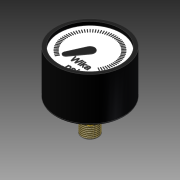
# Autodesk Inventor part: 9690242
Saved by Autodesk Inventor 2014 SP1 (Build 180222100, 222)
## iProperties
Category: Pneumatics
Shininess: 64.0
Length Units: 11269
Angle Units: 11279
Time Units: 11290
Mass Units: 11283
Length Display Precision: 3
Angle Display Precision: 2
Compacted: True
Part Number: 9690242
Document SubType Name: Modeling
Created: 2005-01-09
Manufacturer: Standard
Standards Organization: Custom
Catalog Web Link: www.wika.com
Description: Pressure Gauge
Vendor: WIKA
Density: 1 g/cm^3
Project: FIRST
Material: Generic
Appearance: Glossy - Black
Mass: 32.8384 g
Surface Area: 68.6686 cm^2
Volume: 32.8384 cm^3
Density: 0.0
Volumn: 0.0
Area: 0.0
PropertySet Name: Model Information
Control State: 0
Master: False
Checked Out: False
Title: Pressure Gauge
Author: Autodesk, Inc.
Autodesk Inventor part; units mm, degrees
ref_plane "YZ Plane" through (0, 0, 0) normal (1, 0, 0) x (0, 1, 0)
ref_plane "XZ Plane" through (0, 0, 0) normal (0, 1, 0) x (-1, 0, 0)
ref_plane "XY Plane" through (0, 0, 0) normal (0, 0, 1) x (1, 0, 0)
sketch "Sketch13" plane through (0, 0, 0) normal (0, 0, 1) x (1, 0, 0)
  circle A0 centre (0, 0) radius 20
  dimension "d46" = 40
  constraints: 1 centre point, 1 coincident
  measures "d46" diameter of A0
extrude "Extrusion13" add sketch "Sketch13" along normal blind 26
sketch "Sketch15" plane through (0, 0, 0) normal (0, 0, -1) x (-1, 0, 0)
  line L0 (-7, 7) -> (7, 7)
  line L1 (7, 7) -> (7, -7)
  line L2 (7, -7) -> (-7, -7)
  line L3 (-7, -7) -> (-7, 7)
  line L4 (-28, 0) -> (28, 0) projected
  line L5 (0, -28) -> (0, 28) projected
  dimension "d52" = 14
  dimension "d53" = 14
  constraints: 8 end point, 2 parallel, 1 horizontal, 1 perpendicular, 2 other
  measures "d52" distance of L2.end L0.start
  measures "d53" distance of L0.start L0.end
extrude "Extrusion15" add sketch "Sketch15" along normal blind 8
sketch "Sketch16" plane through (0, 0, -8) normal (0, 0, -1) x (-1, 0, 0)
  circle A0 centre (0, 0) radius 4.7625
  dimension "d58" = 9.525
  constraints: 1 centre point, 1 coincident
  measures "d58" diameter of A0
extrude "Extrusion16" add sketch "Sketch16" along normal blind 10
thread "Thread3" size "1/8" designation "1/8 - 27 NPT" standard "NPT" full length
sketch "Sketch18" plane through (0, 0, 26) normal (0, 0, 1) x (1, 0, 0)
  circle A0 centre (0, 0) radius 20 projected
  circle A1 centre (0, 0) radius 18
  dimension "d66" = 2
  constraints: 1 centre point
  measures "d66" radial gap between concentric circles of A0 A1
extrude "Extrusion18" cut sketch "Sketch18" against normal blind 2 contours A1
sketch "Sketch20" plane through (0, 0, -18) normal (0, 0, -1) x (-1, 0, 0)
  circle A0 centre (0, 0) radius 4.7625 projected
  circle A1 centre (0, 0) radius 1.5
  dimension "d75" = 3
  constraints: 1 centre point, 1 coincident
  measures "d75" diameter of A1
extrude "Extrusion19" cut sketch "Sketch20" against normal blind 10 contours A1
sketch "Sketch19" plane through (0, 0, 24) normal (0, 0, 1) x (1, 0, 0)
  line L0 (-6.3869, -7.2966) -> (14.5094, -7.2966) construction
  line L1 (14.5094, -7.2966) -> (14.5094, -16.6783) construction
  line L2 (14.5094, -16.6783) -> (-6.3869, -16.6783) construction
  line L3 (-6.3869, -16.6783) -> (-6.3869, -7.2966) construction
  circle A0 centre (0, 0) radius 18 projected
  circle A1 centre (0, 0) radius 15 construction
  line L4 (0, 0) -> (-6.5, -11.2583) construction
  line L5 (0, 0) -> (15, 0) construction
  line L6 (-7.6083, -12.9279) -> (-6.6083, -11.1958)
  line L7 (-6.6083, -11.1958) -> (-6.3917, -11.3208)
  line L8 (-6.3917, -11.3208) -> (-7.3917, -13.0529)
  line L9 (-7.3917, -13.0529) -> (-7.6083, -12.9279)
  line L10 (-8.6155, -12.2796) -> (-7.4805, -10.6329)
  line L11 (-7.4805, -10.6329) -> (-7.2746, -10.7748)
  line L12 (-7.2746, -10.7748) -> (-8.4096, -12.4215)
  line L13 (-8.4096, -12.4215) -> (-8.6155, -12.2796)
  line L14 (-9.5677, -11.5531) -> (-8.305, -10.0022)
  line L15 (-8.305, -10.0022) -> (-8.1111, -10.16)
  line L16 (-8.1111, -10.16) -> (-9.3739, -11.7109)
  line L17 (-9.3739, -11.7109) -> (-9.5677, -11.5531)
  line L18 (-10.459, -10.7529) -> (-9.0765, -9.3076)
  line L19 (-9.0765, -9.3076) -> (-8.8959, -9.4805)
  line L20 (-8.8959, -9.4805) -> (-10.2784, -10.9257)
  line L21 (-10.2784, -10.9257) -> (-10.459, -10.7529)
  line L22 (-11.2836, -9.8841) -> (-9.7902, -8.5538)
  line L23 (-9.7902, -8.5538) -> (-9.6239, -8.7405)
  line L24 (-9.6239, -8.7405) -> (-11.1173, -10.0708)
  line L25 (-11.1173, -10.0708) -> (-11.2836, -9.8841)
  line L26 (-12.0362, -8.9523) -> (-10.4415, -7.7454)
  line L27 (-10.4415, -7.7454) -> (-10.2906, -7.9448)
  line L28 (-10.2906, -7.9448) -> (-11.8854, -9.1517)
  line L29 (-11.8854, -9.1517) -> (-12.0362, -8.9523)
  line L30 (-12.7121, -7.9635) -> (-11.0262, -6.8876)
  line L31 (-11.0262, -6.8876) -> (-10.8917, -7.0984)
  line L32 (-10.8917, -7.0984) -> (-12.5777, -8.1742)
  line L33 (-12.5777, -8.1742) -> (-12.7121, -7.9635)
  line L34 (-13.307, -6.9238) -> (-11.5405, -5.9859)
  line L35 (-11.5405, -5.9859) -> (-11.4233, -6.2067)
  line L36 (-11.4233, -6.2067) -> (-13.1898, -7.1446)
  line L37 (-13.1898, -7.1446) -> (-13.307, -6.9238)
  line L38 (-13.817, -5.84) -> (-11.9813, -5.0461)
  line L39 (-11.9813, -5.0461) -> (-11.8821, -5.2755)
  line L40 (-11.8821, -5.2755) -> (-13.7178, -6.0695)
  line L41 (-13.7178, -6.0695) -> (-13.817, -5.84)
  line L42 (-14.2389, -4.719) -> (-12.3458, -4.074)
  line L43 (-12.3458, -4.074) -> (-12.2651, -4.3107)
  line L44 (-12.2651, -4.3107) -> (-14.1583, -4.9557)
  line L45 (-14.1583, -4.9557) -> (-14.2389, -4.719)
  line L46 (-14.57, -3.5679) -> (-12.6315, -3.076)
  line L47 (-12.6315, -3.076) -> (-12.57, -3.3184)
  line L48 (-12.57, -3.3184) -> (-14.5085, -3.8102)
  line L49 (-14.5085, -3.8102) -> (-14.57, -3.5679)
  line L50 (-14.8082, -2.3941) -> (-12.8366, -2.0584)
  line L51 (-12.8366, -2.0584) -> (-12.7947, -2.3049)
  line L52 (-12.7947, -2.3049) -> (-14.7663, -2.6405)
  line L53 (-14.7663, -2.6405) -> (-14.8082, -2.3941)
  line L54 (-14.952, -1.2049) -> (-12.9599, -1.0277)
  line L55 (-12.9599, -1.0277) -> (-12.9378, -1.2767)
  line L56 (-12.9378, -1.2767) -> (-14.9299, -1.4539)
  line L57 (-14.9299, -1.4539) -> (-14.952, -1.2049)
  line L58 (-15.0005, -0.0081) -> (-13.0006, 0.0096)
  line L59 (-13.0006, 0.0096) -> (-12.9984, -0.2404)
  line L60 (-12.9984, -0.2404) -> (-14.9983, -0.2581)
  line L61 (-14.9983, -0.2581) -> (-15.0005, -0.0081)
  line L62 (-14.9533, 1.1887) -> (-12.9584, 1.0469)
  line L63 (-12.9584, 1.0469) -> (-12.9761, 0.7975)
  line L64 (-12.9761, 0.7975) -> (-14.9711, 0.9394)
  line L65 (-14.9711, 0.9394) -> (-14.9533, 1.1887)
  line L66 (-14.8108, 2.378) -> (-12.8335, 2.0774)
  line L67 (-12.8335, 2.0774) -> (-12.8711, 1.8303)
  line L68 (-12.8711, 1.8303) -> (-14.8484, 2.1309)
  line L69 (-14.8484, 2.1309) -> (-14.8108, 2.378)
  line L70 (-14.5739, 3.5521) -> (-12.6269, 3.0947)
  line L71 (-12.6269, 3.0947) -> (-12.6841, 2.8514)
  line L72 (-12.6841, 2.8514) -> (-14.6311, 3.3088)
  line L73 (-14.6311, 3.3088) -> (-14.5739, 3.5521)
  line L74 (-14.244, 4.7036) -> (-12.3397, 4.0923)
  line L75 (-12.3397, 4.0923) -> (-12.4161, 3.8543)
  line L76 (-12.4161, 3.8543) -> (-14.3204, 4.4656)
  line L77 (-14.3204, 4.4656) -> (-14.244, 4.7036)
  line L78 (-13.8233, 5.8251) -> (-11.9739, 5.0638)
  line L79 (-11.9739, 5.0638) -> (-12.069, 4.8326)
  line L80 (-12.069, 4.8326) -> (-13.9185, 5.5939)
  line L81 (-13.9185, 5.5939) -> (-13.8233, 5.8251)
  line L82 (-13.3145, 6.9094) -> (-11.5317, 6.003)
  line L83 (-11.5317, 6.003) -> (-11.645, 5.7802)
  line L84 (-11.645, 5.7802) -> (-13.4278, 6.6866)
  line L85 (-13.4278, 6.6866) -> (-13.3145, 6.9094)
  line L86 (-12.7208, 7.9497) -> (-11.0159, 6.904)
  line L87 (-11.0159, 6.904) -> (-11.1467, 6.6908)
  line L88 (-11.1467, 6.6908) -> (-12.8515, 7.7366)
  line L89 (-12.8515, 7.7366) -> (-12.7208, 7.9497)
  line L90 (-12.0459, 8.9393) -> (-10.43, 7.7609)
  line L91 (-10.43, 7.7609) -> (-10.5773, 7.5589)
  line L92 (-10.5773, 7.5589) -> (-12.1932, 8.7373)
  line L93 (-12.1932, 8.7373) -> (-12.0459, 8.9393)
  line L94 (-11.2943, 9.8719) -> (-9.7775, 8.5683)
  line L95 (-9.7775, 8.5683) -> (-9.9405, 8.3787)
  line L96 (-9.9405, 8.3787) -> (-11.4573, 9.6823)
  line L97 (-11.4573, 9.6823) -> (-11.2943, 9.8719)
  line L98 (-10.4707, 10.7416) -> (-9.0627, 9.3211)
  line L99 (-9.0627, 9.3211) -> (-9.2403, 9.1451)
  line L100 (-9.2403, 9.1451) -> (-10.6482, 10.5656)
  line L101 (-10.6482, 10.5656) -> (-10.4707, 10.7416)
  line L102 (-9.5802, 11.5427) -> (-8.2901, 10.0144)
  line L103 (-8.2901, 10.0144) -> (-8.4812, 9.8532)
  line L104 (-8.4812, 9.8532) -> (-9.7713, 11.3815)
  line L105 (-9.7713, 11.3815) -> (-9.5802, 11.5427)
  line L106 (-8.6288, 12.2703) -> (-7.4647, 10.644)
  line L107 (-7.4647, 10.644) -> (-7.668, 10.4985)
  line L108 (-7.668, 10.4985) -> (-8.832, 12.1248)
  line L109 (-8.832, 12.1248) -> (-8.6288, 12.2703)
  line L110 (-7.6222, 12.9196) -> (-6.5917, 11.2056)
  line L111 (-6.5917, 11.2056) -> (-6.8059, 11.0768)
  line L112 (-6.8059, 11.0768) -> (-7.8365, 12.7908)
  line L113 (-7.8365, 12.7908) -> (-7.6222, 12.9196)
  line L114 (-6.5671, 13.4866) -> (-5.6766, 11.6958)
  line L115 (-5.6766, 11.6958) -> (-5.9004, 11.5845)
  line L116 (-5.9004, 11.5845) -> (-6.791, 13.3753)
  line L117 (-6.791, 13.3753) -> (-6.5671, 13.4866)
  line L118 (-5.4702, 13.9676) -> (-4.7253, 12.1114)
  line L119 (-4.7253, 12.1114) -> (-4.9574, 12.0183)
  line L120 (-4.9574, 12.0183) -> (-5.7022, 13.8745)
  line L121 (-5.7022, 13.8745) -> (-5.4702, 13.9676)
  line L122 (-4.3383, 14.3595) -> (-3.744, 12.4498)
  line L123 (-3.744, 12.4498) -> (-3.9827, 12.3755)
  line L124 (-3.9827, 12.3755) -> (-4.577, 14.2852)
  line L125 (-4.577, 14.2852) -> (-4.3383, 14.3595)
  line L126 (-3.1788, 14.6598) -> (-2.7387, 12.7089)
  line L127 (-2.7387, 12.7089) -> (-2.9826, 12.6539)
  line L128 (-2.9826, 12.6539) -> (-3.4227, 14.6048)
  line L129 (-3.4227, 14.6048) -> (-3.1788, 14.6598)
  line L130 (-1.999, 14.8667) -> (-1.716, 12.8869)
  line L131 (-1.716, 12.8869) -> (-1.9635, 12.8515)
  line L132 (-1.9635, 12.8515) -> (-2.2465, 14.8313)
  line L133 (-2.2465, 14.8313) -> (-1.999, 14.8667)
  line L134 (-0.8065, 14.9788) -> (-0.6823, 12.9827)
  line L135 (-0.6823, 12.9827) -> (-0.9318, 12.9672)
  line L136 (-0.9318, 12.9672) -> (-1.056, 14.9633)
  line L137 (-1.056, 14.9633) -> (-0.8065, 14.9788)
  line L138 (0.3912, 14.9954) -> (0.3557, 12.9957)
  line L139 (0.3557, 12.9957) -> (0.1057, 13.0002)
  line L140 (0.1057, 13.0002) -> (0.1412, 14.9999)
  line L141 (0.1412, 14.9999) -> (0.3912, 14.9954)
  line L142 (1.5864, 14.9164) -> (1.3915, 12.9259)
  line L143 (1.3915, 12.9259) -> (1.1426, 12.9503)
  line L144 (1.1426, 12.9503) -> (1.3376, 14.9408)
  line L145 (1.3376, 14.9408) -> (1.5864, 14.9164)
  line L146 (2.7714, 14.7423) -> (2.4183, 12.7737)
  line L147 (2.4183, 12.7737) -> (2.1723, 12.8178)
  line L148 (2.1723, 12.8178) -> (2.5254, 14.7864)
  line L149 (2.5254, 14.7864) -> (2.7714, 14.7423)
  line L150 (3.9388, 14.4742) -> (3.4298, 12.54)
  line L151 (3.4298, 12.54) -> (3.188, 12.6037)
  line L152 (3.188, 12.6037) -> (3.6971, 14.5378)
  line L153 (3.6971, 14.5378) -> (3.9388, 14.4742)
  line L154 (5.0811, 14.1137) -> (4.4194, 12.2264)
  line L155 (4.4194, 12.2264) -> (4.1834, 12.3091)
  line L156 (4.1834, 12.3091) -> (4.8452, 14.1965)
  line L157 (4.8452, 14.1965) -> (5.0811, 14.1137)
  line L158 (6.191, 13.6633) -> (5.3808, 11.8348)
  line L159 (5.3808, 11.8348) -> (5.1522, 11.9361)
  line L160 (5.1522, 11.9361) -> (5.9624, 13.7646)
  line L161 (5.9624, 13.7646) -> (6.191, 13.6633)
  line L162 (7.2614, 13.1258) -> (6.3079, 11.3678)
  line L163 (6.3079, 11.3678) -> (6.0881, 11.487)
  line L164 (6.0881, 11.487) -> (7.0417, 13.245)
  line L165 (7.0417, 13.245) -> (7.2614, 13.1258)
  line L166 (8.2855, 12.5046) -> (7.1948, 10.8283)
  line L167 (7.1948, 10.8283) -> (6.9852, 10.9646)
  line L168 (6.9852, 10.9646) -> (8.076, 12.641)
  line L169 (8.076, 12.641) -> (8.2855, 12.5046)
  line L170 (9.2568, 11.8037) -> (8.0358, 10.2197)
  line L171 (8.0358, 10.2197) -> (7.8378, 10.3723)
  line L172 (7.8378, 10.3723) -> (9.0588, 11.9563)
  line L173 (9.0588, 11.9563) -> (9.2568, 11.8037)
  line L174 (10.1691, 11.0275) -> (8.8255, 9.546)
  line L175 (8.8255, 9.546) -> (8.6403, 9.7139)
  line L176 (8.6403, 9.7139) -> (9.9839, 11.1954)
  line L177 (9.9839, 11.1954) -> (10.1691, 11.0275)
  line L178 (11.0165, 10.181) -> (9.559, 8.8114)
  line L179 (9.559, 8.8114) -> (9.3878, 8.9936)
  line L180 (9.3878, 8.9936) -> (10.8453, 10.3632)
  line L181 (10.8453, 10.3632) -> (11.0165, 10.181)
  line L182 (11.7937, 9.2696) -> (10.2316, 8.0206)
  line L183 (10.2316, 8.0206) -> (10.0755, 8.2159)
  line L184 (10.0755, 8.2159) -> (11.6375, 9.4648)
  line L185 (11.6375, 9.4648) -> (11.7937, 9.2696)
  line L186 (12.4957, 8.2991) -> (10.8389, 7.1787)
  line L187 (10.8389, 7.1787) -> (10.6989, 7.3858)
  line L188 (10.6989, 7.3858) -> (12.3556, 8.5061)
  line L189 (12.3556, 8.5061) -> (12.4957, 8.2991)
  line L190 (13.118, 7.2756) -> (11.3771, 6.291)
  line L191 (11.3771, 6.291) -> (11.254, 6.5086)
  line L192 (11.254, 6.5086) -> (12.9949, 7.4932)
  line L193 (12.9949, 7.4932) -> (13.118, 7.2756)
  line L194 (13.6566, 6.2058) -> (11.8428, 5.3632)
  line L195 (11.8428, 5.3632) -> (11.7375, 5.59)
  line L196 (11.7375, 5.59) -> (13.5513, 6.4325)
  line L197 (13.5513, 6.4325) -> (13.6566, 6.2058)
  line L198 (14.1082, 5.0964) -> (12.2329, 4.4013)
  line L199 (12.2329, 4.4013) -> (12.146, 4.6357)
  line L200 (12.146, 4.6357) -> (14.0213, 5.3308)
  line L201 (14.0213, 5.3308) -> (14.1082, 5.0964)
  line L202 (14.4699, 3.9545) -> (12.5451, 3.4112)
  line L203 (12.5451, 3.4112) -> (12.4772, 3.6518)
  line L204 (12.4772, 3.6518) -> (14.402, 4.1951)
  line L205 (14.402, 4.1951) -> (14.4699, 3.9545)
  line L206 (-6.6396, -8.3604) -> (-2.4534, 1.0871)
  arc A2 (2.1681, -1.5811) -> (-2.4534, 1.0871) centre (0, 0) ccw
  line L207 (14.7393, 2.7874) -> (12.7773, 2.3994)
  line L208 (12.7773, 2.3994) -> (12.7288, 2.6447)
  line L209 (12.7288, 2.6447) -> (14.6908, 3.0327)
  line L210 (14.6908, 3.0327) -> (14.7393, 2.7874)
  line L211 (14.9147, 1.6025) -> (12.928, 1.3723)
  line L212 (12.928, 1.3723) -> (12.8992, 1.6206)
  line L213 (12.8992, 1.6206) -> (14.8859, 1.8509)
  line L214 (14.8859, 1.8509) -> (14.9147, 1.6025)
  line L215 (14.995, 0.4074) -> (12.9962, 0.3365)
  line L216 (12.9962, 0.3365) -> (12.9874, 0.5863)
  line L217 (12.9874, 0.5863) -> (14.9861, 0.6573)
  line L218 (14.9861, 0.6573) -> (14.995, 0.4074)
  line L219 (14.9797, -0.7903) -> (12.9817, -0.7015)
  line L220 (12.9817, -0.7015) -> (12.9927, -0.4518)
  line L221 (12.9927, -0.4518) -> (14.9908, -0.5405)
  line L222 (14.9908, -0.5405) -> (14.9797, -0.7903)
  line L223 (14.8689, -1.9829) -> (12.8843, -1.7351)
  line L224 (12.8843, -1.7351) -> (12.9153, -1.487)
  line L225 (12.9153, -1.487) -> (14.8999, -1.7348)
  line L226 (14.8999, -1.7348) -> (14.8689, -1.9829)
  line L227 (14.6633, -3.1629) -> (12.7048, -2.7575)
  line L228 (12.7048, -2.7575) -> (12.7555, -2.5127)
  line L229 (12.7555, -2.5127) -> (14.7139, -2.9181)
  line L230 (14.7139, -2.9181) -> (14.6633, -3.1629)
  line L231 (14.3642, -4.3228) -> (12.4443, -3.7624)
  line L232 (12.4443, -3.7624) -> (12.5143, -3.5224)
  line L233 (12.5143, -3.5224) -> (14.4342, -4.0828)
  line L234 (14.4342, -4.0828) -> (14.3642, -4.3228)
  line L235 (13.9735, -5.455) -> (12.1044, -4.7433)
  line L236 (12.1044, -4.7433) -> (12.1934, -4.5096)
  line L237 (12.1934, -4.5096) -> (14.0625, -5.2214)
  line L238 (14.0625, -5.2214) -> (13.9735, -5.455)
  line L239 (13.4937, -6.5525) -> (11.6874, -5.6939)
  line L240 (11.6874, -5.6939) -> (11.7947, -5.4681)
  line L241 (11.7947, -5.4681) -> (13.601, -6.3267)
  line L242 (13.601, -6.3267) -> (13.4937, -6.5525)
  line L243 (12.9279, -7.6083) -> (11.1958, -6.6083)
  line L244 (11.1958, -6.6083) -> (11.3208, -6.3917)
  line L245 (11.3208, -6.3917) -> (13.0529, -7.3917)
  line L246 (13.0529, -7.3917) -> (12.9279, -7.6083)
  line L247 (-6.5, -11.2583) -> (-7.5, -12.9904) construction
  line L248 (2.1681, -1.5811) -> (-3.9205, -9.9303)
  arc A3 (-6.6396, -8.3604) -> (-3.9205, -9.9303) centre (-5.1962, -9) ccw
  line L249 (-0.3844, -10.7966) -> (-1.3128, -7.2966)
  line L250 (-1.3128, -7.2966) -> (-0.8379, -7.2966)
  line L251 (-0.8379, -7.2966) -> (-0.3044, -9.5908)
  spline S0 degree 2 poles (-0.3044, -9.5908) (-0.219, -9.951) (-0.155, -10.3084) knots 0 0 0 1 1 1
  spline S1 degree 2 poles (-0.155, -10.3084) (-0.0216, -9.7456) (0.0024, -9.6602) knots 0 0 0 1 1 1
  line L252 (0.0024, -9.6602) -> (0.6666, -7.2966)
  line L253 (0.6666, -7.2966) -> (1.2269, -7.2966)
  line L254 (1.2269, -7.2966) -> (1.7284, -9.068)
  spline S2 degree 2 poles (1.7284, -9.068) (1.9124, -9.7269) (2.0005, -10.3084) knots 0 0 0 1 1 1
  spline S3 degree 2 poles (2.0005, -10.3084) (2.0672, -9.975) (2.1739, -9.5455) knots 0 0 0 1 1 1
  line L255 (2.1739, -9.5455) -> (2.7208, -7.2966)
  line L256 (2.7208, -7.2966) -> (3.1876, -7.2966)
  line L257 (3.1876, -7.2966) -> (2.2326, -10.7966)
  line L258 (2.2326, -10.7966) -> (1.7791, -10.7966)
  line L259 (1.7791, -10.7966) -> (1.0481, -8.1289)
  spline S4 degree 2 poles (1.0481, -8.1289) (0.9521, -7.7955) (0.9361, -7.7181) knots 0 0 0 1 1 1
  spline S5 degree 2 poles (0.9361, -7.7181) (0.8774, -7.9582) (0.832, -8.1289) knots 0 0 0 1 1 1
  line L260 (0.832, -8.1289) -> (0.0931, -10.7966)
  line L261 (0.0931, -10.7966) -> (-0.3844, -10.7966)
  line L262 (3.5691, -10.7966) -> (3.5691, -8.2597)
  line L263 (3.5691, -8.2597) -> (3.9986, -8.2597)
  line L264 (3.9986, -8.2597) -> (3.9986, -10.7966)
  line L265 (3.9986, -10.7966) -> (3.5691, -10.7966)
  line L266 (3.5691, -7.7902) -> (3.5691, -7.2966)
  line L267 (3.5691, -7.2966) -> (3.9986, -7.2966)
  line L268 (3.9986, -7.2966) -> (3.9986, -7.7902)
  line L269 (3.9986, -7.7902) -> (3.5691, -7.7902)
  line L270 (4.6548, -10.7966) -> (4.6548, -7.2966)
  line L271 (4.6548, -7.2966) -> (5.0843, -7.2966)
  line L272 (5.0843, -7.2966) -> (5.0843, -9.2921)
  line L273 (5.0843, -9.2921) -> (6.1007, -8.2597)
  line L274 (6.1007, -8.2597) -> (6.6583, -8.2597)
  line L275 (6.6583, -8.2597) -> (5.6899, -9.2014)
  line L276 (5.6899, -9.2014) -> (6.757, -10.7966)
  line L277 (6.757, -10.7966) -> (6.2261, -10.7966)
  line L278 (6.2261, -10.7966) -> (5.3831, -9.5001)
  line L279 (5.3831, -9.5001) -> (5.0843, -9.7909)
  line L280 (5.0843, -9.7909) -> (5.0843, -10.7966)
  line L281 (5.0843, -10.7966) -> (4.6548, -10.7966)
  spline S6 degree 2 poles (8.7524, -10.4845) (8.5123, -10.6873) (8.0721, -10.8527) (7.8187, -10.8527) knots 0 0 0 1 2 2 2
  spline S7 degree 2 poles (7.8187, -10.8527) (7.3999, -10.8527) (6.9517, -10.4445) (6.9517, -10.127) knots 0 0 0 1 2 2 2
  spline S8 degree 2 poles (6.9517, -10.127) (6.9517, -9.9403) (7.1224, -9.6335) (7.3945, -9.4468) (7.5679, -9.4014) knots 0 0 0 1 2 3 3 3
  spline S9 degree 2 poles (7.5679, -9.4014) (7.6933, -9.3668) (7.9494, -9.3347) knots 0 0 0 1 1 1
  spline S10 degree 2 poles (7.9494, -9.3347) (8.4696, -9.2734) (8.715, -9.188) knots 0 0 0 1 1 1
  spline S11 degree 2 poles (8.715, -9.188) (8.7177, -9.1) (8.7177, -9.076) knots 0 0 0 1 1 1
  spline S12 degree 2 poles (8.7177, -9.076) (8.7177, -8.8119) (8.595, -8.7052) knots 0 0 0 1 1 1
  spline S13 degree 2 poles (8.595, -8.7052) (8.4323, -8.5584) (8.1068, -8.5584) knots 0 0 0 1 1 1
  spline S14 degree 2 poles (8.1068, -8.5584) (7.8054, -8.5584) (7.5173, -8.7719) (7.4479, -9.0413) knots 0 0 0 1 2 2 2
  line L282 (7.4479, -9.0413) -> (7.0264, -8.9853)
  spline S15 degree 2 poles (7.0264, -8.9853) (7.0824, -8.7158) (7.3465, -8.3824) (7.8427, -8.2036) (8.1682, -8.2036) knots 0 0 0 1 2 3 3 3
  spline S16 degree 2 poles (8.1682, -8.2036) (8.4936, -8.2036) (8.8991, -8.3557) (9.0912, -8.5878) (9.1285, -8.7639) knots 0 0 0 1 2 3 3 3
  spline S17 degree 2 poles (9.1285, -8.7639) (9.1499, -8.8759) (9.1499, -9.1613) knots 0 0 0 1 1 1
  line L283 (9.1499, -9.1613) -> (9.1499, -9.7349)
  spline S18 degree 2 poles (9.1499, -9.7349) (9.1499, -10.3325) (9.2059, -10.6499) (9.2859, -10.7966) knots 0 0 0 1 2 2 2
  line L284 (9.2859, -10.7966) -> (8.8378, -10.7966)
  spline S19 degree 2 poles (8.8378, -10.7966) (8.7711, -10.6632) (8.7524, -10.4845) knots 0 0 0 1 1 1
  spline S20 degree 2 poles (8.7177, -9.5241) (8.483, -9.6202) (8.0161, -9.6869) knots 0 0 0 1 1 1
  spline S21 degree 2 poles (8.0161, -9.6869) (7.7493, -9.7242) (7.5306, -9.8203) (7.4105, -10.0043) (7.4105, -10.1164) knots 0 0 0 1 2 3 3 3
  spline S22 degree 2 poles (7.4105, -10.1164) (7.4105, -10.2871) (7.6693, -10.5165) (7.9201, -10.5165) knots 0 0 0 1 2 2 2
  spline S23 degree 2 poles (7.9201, -10.5165) (8.1682, -10.5165) (8.555, -10.3004) (8.6457, -10.111) knots 0 0 0 1 2 2 2
  spline S24 degree 2 poles (8.6457, -10.111) (8.715, -9.9643) (8.715, -9.6815) knots 0 0 0 1 1 1
  line L285 (8.715, -9.6815) -> (8.7177, -9.5241)
  line L286 (1.2589, -17.2756) -> (1.2589, -13.7676)
  line L287 (1.2589, -13.7676) -> (1.651, -13.7676)
  line L288 (1.651, -13.7676) -> (1.651, -14.0984)
  spline S25 degree 2 poles (1.651, -14.0984) (1.7897, -13.9037) (2.1365, -13.7116) (2.3873, -13.7116) knots 0 0 0 1 2 2 2
  spline S26 degree 2 poles (2.3873, -13.7116) (2.7101, -13.7116) (3.2063, -14.0451) (3.4597, -14.6533) (3.4597, -15.0161) knots 0 0 0 1 2 3 3 3
  spline S27 degree 2 poles (3.4597, -15.0161) (3.4597, -15.4056) (3.1796, -16.0298) (2.6487, -16.3606) (2.3553, -16.3606) knots 0 0 0 1 2 3 3 3
  spline S28 degree 2 poles (2.3553, -16.3606) (2.1392, -16.3606) (1.7977, -16.1792) (1.6884, -16.0405) knots 0 0 0 1 2 2 2
  line L289 (1.6884, -16.0405) -> (1.6884, -17.2756)
  line L290 (1.6884, -17.2756) -> (1.2589, -17.2756)
  spline S29 degree 2 poles (1.6483, -15.0508) (1.6483, -15.5416) (2.0432, -16.0085) (2.3233, -16.0085) knots 0 0 0 1 2 2 2
  spline S30 degree 2 poles (2.3233, -16.0085) (2.6087, -16.0085) (3.0169, -15.523) (3.0169, -15.0161) knots 0 0 0 1 2 2 2
  spline S31 degree 2 poles (3.0169, -15.0161) (3.0169, -14.5306) (2.6194, -14.0477) (2.3446, -14.0477) knots 0 0 0 1 2 2 2
  spline S32 degree 2 poles (2.3446, -14.0477) (2.0698, -14.0477) (1.6483, -14.5599) (1.6483, -15.0508) knots 0 0 0 1 2 2 2
  line L291 (3.8038, -15.547) -> (4.228, -15.4803)
  spline S33 degree 2 poles (4.228, -15.4803) (4.2627, -15.7364) (4.5908, -16.0085) (4.8869, -16.0085) knots 0 0 0 1 2 2 2
  spline S34 degree 2 poles (4.8869, -16.0085) (5.183, -16.0085) (5.4711, -15.7657) (5.4711, -15.603) knots 0 0 0 1 2 2 2
  spline S35 degree 2 poles (5.4711, -15.603) (5.4711, -15.4589) (5.3431, -15.3736) knots 0 0 0 1 1 1
  spline S36 degree 2 poles (5.3431, -15.3736) (5.2551, -15.3175) (4.9029, -15.2295) knots 0 0 0 1 1 1
  spline S37 degree 2 poles (4.9029, -15.2295) (4.4307, -15.1095) (4.0653, -14.9361) (3.8759, -14.6266) (3.8759, -14.4425) knots 0 0 0 1 2 3 3 3
  spline S38 degree 2 poles (3.8759, -14.4425) (3.8759, -14.2718) (4.0306, -13.9837) (4.164, -13.8877) knots 0 0 0 1 2 2 2
  spline S39 degree 2 poles (4.164, -13.8877) (4.2653, -13.813) (4.6121, -13.7116) (4.8122, -13.7116) knots 0 0 0 1 2 2 2
  spline S40 degree 2 poles (4.8122, -13.7116) (5.111, -13.7116) (5.5618, -13.885) (5.7779, -14.1784) (5.8179, -14.4239) knots 0 0 0 1 2 3 3 3
  line L292 (5.8179, -14.4239) -> (5.3964, -14.4799)
  spline S41 degree 2 poles (5.3964, -14.4799) (5.3671, -14.2825) (5.0923, -14.0637) (4.8416, -14.0637) knots 0 0 0 1 2 2 2
  spline S42 degree 2 poles (4.8416, -14.0637) (4.5455, -14.0637) (4.292, -14.2611) (4.292, -14.3919) knots 0 0 0 1 2 2 2
  spline S43 degree 2 poles (4.292, -14.3919) (4.292, -14.4746) (4.3454, -14.5413) knots 0 0 0 1 1 1
  spline S44 degree 2 poles (4.3454, -14.5413) (4.3961, -14.6106) (4.5108, -14.656) knots 0 0 0 1 1 1
  spline S45 degree 2 poles (4.5108, -14.656) (4.5748, -14.68) (4.8896, -14.768) knots 0 0 0 1 1 1
  spline S46 degree 2 poles (4.8896, -14.768) (5.3458, -14.888) (5.7086, -15.0428) (5.914, -15.3389) (5.914, -15.5603) knots 0 0 0 1 2 3 3 3
  spline S47 degree 2 poles (5.914, -15.5603) (5.914, -15.7737) (5.6632, -16.1525) (5.1884, -16.3606) (4.8896, -16.3606) knots 0 0 0 1 2 3 3 3
  spline S48 degree 2 poles (4.8896, -16.3606) (4.3961, -16.3606) (3.8759, -15.9498) (3.8038, -15.547) knots 0 0 0 1 2 2 2
  line L293 (6.4262, -16.3046) -> (6.4262, -13.7676)
  line L294 (6.4262, -13.7676) -> (6.8557, -13.7676)
  line L295 (6.8557, -13.7676) -> (6.8557, -16.3046)
  line L296 (6.8557, -16.3046) -> (6.4262, -16.3046)
  line L297 (6.4262, -13.2981) -> (6.4262, -12.8046)
  line L298 (6.4262, -12.8046) -> (6.8557, -12.8046)
  line L299 (6.8557, -12.8046) -> (6.8557, -13.2981)
  line L300 (6.8557, -13.2981) -> (6.4262, -13.2981)
  point P0 (-7.3775, -10.7038)
  point P1 (-8.5125, -12.3506)
  point P2 (-8.208, -10.0811)
  point P3 (-9.4708, -11.632)
  point P4 (-8.9862, -9.3941)
  point P5 (-10.3687, -10.8393)
  point P6 (-9.7071, -8.6471)
  point P7 (-11.2005, -9.9775)
  point P8 (-10.366, -7.8451)
  point P9 (-11.9608, -9.052)
  point P10 (-10.9589, -6.993)
  point P11 (-12.6449, -8.0688)
  point P12 (-11.4819, -6.0963)
  point P13 (-13.2484, -7.0342)
  point P14 (-11.9317, -5.1608)
  point P15 (-13.7674, -5.9548)
  point P16 (-12.3054, -4.1924)
  point P17 (-14.1986, -4.8373)
  point P18 (-12.6007, -3.1972)
  point P19 (-14.5393, -3.6891)
  point P20 (-12.8156, -2.1816)
  point P21 (-14.7873, -2.5173)
  point P22 (-12.9488, -1.1522)
  point P23 (-14.941, -1.3294)
  point P24 (-12.9995, -0.1154)
  point P25 (-14.9994, -0.1331)
  point P26 (-12.9673, 0.9222)
  point P27 (-14.9622, 1.0641)
  point P28 (-12.8523, 1.9538)
  point P29 (-14.8296, 2.2544)
  point P30 (-12.6555, 2.9731)
  point P31 (-14.6025, 3.4304)
  point P32 (-12.3779, 3.9733)
  point P33 (-14.2822, 4.5846)
  point P34 (-12.0214, 4.9482)
  point P35 (-13.8709, 5.7095)
  point P36 (-11.5883, 5.8916)
  point P37 (-13.3711, 6.798)
  point P38 (-11.0813, 6.7974)
  point P39 (-12.7861, 7.8432)
  point P40 (-10.5036, 7.6599)
  point P41 (-12.1196, 8.8383)
  point P42 (-9.859, 8.4735)
  point P43 (-11.3758, 9.7771)
  point P44 (-9.1515, 9.2331)
  point P45 (-10.5594, 10.6536)
  point P46 (-8.3857, 9.9338)
  point P47 (-9.6758, 11.4621)
  point P48 (-7.5663, 10.5712)
  point P49 (-8.7304, 12.1975)
  point P50 (-6.6988, 11.1412)
  point P51 (-7.7294, 12.8552)
  point P52 (-5.7885, 11.6401)
  point P53 (-6.6791, 13.4309)
  point P54 (-4.8413, 12.0649)
  point P55 (-5.5862, 13.921)
  point P56 (-3.8633, 12.4127)
  point P57 (-4.4577, 14.3223)
  point P58 (-2.8606, 12.6814)
  point P59 (-3.3007, 14.6323)
  point P60 (-1.8397, 12.8692)
  point P61 (-2.1227, 14.849)
  point P62 (-0.8071, 12.9749)
  point P63 (-0.9312, 14.9711)
  point P64 (0.2307, 12.998)
  point P65 (0.2662, 14.9976)
  point P66 (1.267, 12.9381)
  point P67 (1.462, 14.9286)
  point P68 (2.2953, 12.7958)
  point P69 (2.6484, 14.7643)
  point P70 (3.3089, 12.5718)
  point P71 (3.818, 14.506)
  point P72 (4.3014, 12.2678)
  point P73 (4.9632, 14.1551)
  point P74 (5.2665, 11.8855)
  point P75 (6.0767, 13.714)
  point P76 (6.198, 11.4274)
  point P77 (7.1515, 13.1854)
  point P78 (7.09, 10.8964)
  point P79 (8.1807, 12.5728)
  point P80 (7.9368, 10.296)
  point P81 (9.1578, 11.88)
  point P82 (8.7329, 9.6299)
  point P83 (10.0765, 11.1115)
  point P84 (9.4734, 8.9025)
  point P85 (10.9309, 10.2721)
  point P86 (10.1535, 8.1182)
  point P87 (11.7156, 9.3672)
  point P88 (10.7689, 7.2823)
  point P89 (12.4256, 8.4026)
  point P90 (11.3156, 6.3998)
  point P91 (13.0564, 7.3844)
  point P92 (11.7901, 5.4766)
  point P93 (13.604, 6.3192)
  point P94 (12.1895, 4.5185)
  point P95 (14.0648, 5.2136)
  point P96 (12.5111, 3.5315)
  point P97 (14.4359, 4.0748)
  point P98 (-12.6228, -21.8633)
  point P99 (12.753, 2.522)
  point P100 (14.715, 2.91)
  point P101 (12.9136, 1.4965)
  point P102 (14.9003, 1.7267)
  point P103 (12.9918, 0.4614)
  point P104 (14.9906, 0.5324)
  point P105 (12.9872, -0.5767)
  point P106 (14.9852, -0.6654)
  point P107 (12.8998, -1.611)
  point P108 (14.8844, -1.8589)
  point P109 (12.7301, -2.6351)
  point P110 (14.6886, -3.0405)
  point P111 (12.4793, -3.6424)
  point P112 (14.3992, -4.2028)
  point P113 (12.1489, -4.6265)
  point P114 (14.018, -5.3382)
  point P115 (11.741, -5.581)
  point P116 (13.5474, -6.4396)
  point P117 (11.2583, -6.5)
  point P118 (12.9904, -7.5)
  dimension "d76" = 30
  dimension "d77" = 120
  dimension "d78" = 0.25
  dimension "d79" = 2
  dimension "d82" = 270
  dimension "d87" = 2.6834
  dimension "d91" = 9
  constraints: 490 end point, 6 point on circle, 5 parallel, 4 tangent, 3 centre point, 3 midpoint, 3 point on line, 2 coincident, 1 horizontal, 1 perpendicular, 593 other
  measures "d76" diameter of A1
  measures "d77" angle of L5 L4
  measures "d78" distance of L6.end L7.end
  measures "d79" distance of L7.end L8.end
  measures "d87" radius of A2
  measures "d91" distance from line of L5 A3.centre
chamfer "Chamfer1" distance 0.5 angle 45 1 edges at (4.7625, 0, -18)
fillet "Fillet5" radius 1 1 edges at (-20, 0, 0)
extrude "Extrusion20" add sketch "Sketch19" along normal blind 0.2 contours L6 L7 L8 L9 | L10 L11 L12 L13 | L14 L15 L16 L17 | L18 L19 L20 L21 | L22 L23 L24 L25 | L26 L27 L28 L29 | L30 L31 L32 L33 | L34 L35 L36 L37 | L38 L39 L40 L41 | L42 L43 L44 L45 | L46 L47 L48 L49 | L50 L51 L52 L53 | L54 L55 L56 L57 | L58 L59 L60 L61 | L62 L63 L64 L65 | L66 L67 L68 L69 | L70 L71 L72 L73 | L74 L75 L76 L77 | L78 L79 L80 L81 | L82 L83 L84 L85 | L86 L87 L88 L89 | L90 L91 L92 L93 | L94 L95 L96 L97 | L98 L99 L100 L101 | L102 L103 L104 L105 | L106 L107 L108 L109 | L110 L111 L112 L113 | L114 L115 L116 L117 | L118 L119 L120 L121 | L122 L123 L124 L125 | L126 L127 L128 L129 | L130 L131 L132 L133 | L134 L135 L136 L137 | L138 L139 L140 L141 | L142 L143 L144 L145 | L146 L147 L148 L149 | L150 L151 L152 L153 | L154 L155 L156 L157 | L158 L159 L160 L161 | L162 L163 L164 L165 | L166 L167 L168 L169 | L170 L171 L172 L173 | L174 L175 L176 L177 | L178 L179 L180 L181 | L182 L183 L184 L185 | L186 L187 L188 L189 | L190 L191 L192 L193 | L194 L195 L196 L197 | L198 L199 L200 L201 | L202 L203 L204 L205 | L206 A2 L248 A3 | L207 L208 L209 L210 | L211 L212 L213 L214 | L215 L216 L217 L218 | L219 L220 L221 L222 | L223 L224 L225 L226 | L227 L228 L229 L230 | L231 L232 L233 L234 | L235 L236 L237 L238 | L239 L240 L241 L242 | L243 L244 L245 L246 | L249 L250 L251 S0 S1 L252 L253 L254 S2 S3 L255 L256 L257 L258 L259 S4 S5 L260 L261 | L262 L263 L264 L265 | L266 L267 L268 L269 | L270 L271 L272 L273 L274 L275 L276 L277 L278 L279 L280 L281 | S6 S7 S8 S9 S10 S11 S12 S13 S14 L282 S15 S16 S17 L283 S18 L284 S19 | L286 L287 L288 S25 S26 S27 S28 L289 L290 | L291 S33 S34 S35 S36 S37 S38 S39 S40 L292 S41 S42 S43 S44 S45 S46 S47 S48 | L293 L294 L295 L296 | L297 L298 L299 L300
body "Solid1"
